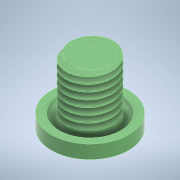
# Autodesk Inventor part: screw_oring
Saved by Autodesk Inventor 2022 (Build 260153000, 153)
## iProperties
Created: 2022-10-25
Part Number: screw_oring
Material: Ogólny
Document SubType Name: Modeling
Designer: kosak
Density: 1 g/cm^3
Appearance: Gładki — ciemna zieleń leśna
Author: kosak
Autodesk Inventor part; units mm, degrees
ref_plane "YZ Plane" through (0, 0, 0) normal (1, 0, 0) x (0, 1, 0)
ref_plane "XZ Plane" through (0, 0, 0) normal (0, 1, 0) x (-1, 0, 0)
ref_plane "XY Plane" through (0, 0, 0) normal (0, 0, 1) x (1, 0, 0)
sketch "Szkic1" plane through (0, 0, 0) normal (0, 1, 0) x (-1, 0, 0)
  circle A0 centre (0, 0) radius 11.5
  dimension "d0" = 23
  constraints: 1 centre point, 1 coincident
  measures "d0" diameter of A0
extrude "Wyciągnięcie proste1" add sketch "Szkic1" along normal blind 4
sketch "Szkic2" plane through (0, 4, 0) normal (0, 1, 0) x (1, 0, 0)
  circle A0 centre (0, 0) radius 6.85
  circle A1 centre (0, 0) radius 9.15
  dimension "d3" = 13.7
  dimension "d4" = 18.3
  constraints: 2 centre point, 2 coincident
  measures "d3" diameter of A0
  measures "d4" diameter of A1
extrude "Wyciągnięcie proste2" cut sketch "Szkic2" against normal blind 1.5
sketch "Szkic3" plane through (0, 4, 0) normal (0, 1, 0) x (1, 0, 0)
  circle A0 centre (0, 0) radius 7
  dimension "d8" = 14
  constraints: 1 centre point, 1 coincident
  measures "d8" diameter of A0
extrude "Wyciągnięcie proste3" add sketch "Szkic3" along normal blind 15
thread "Gwint1" size "M14x2" class "6g" standard "ANSI Metric M Profile" full length
full round fillet "Zaokrąglenie pełne3" first side at (9.1203, 3, 0.7363) centre faces at (8.2947, 2.5, 0.7299) second side at (6.8278, 3, 0.5512)
sketch "Szkic5" plane through (0, 19, 0) normal (1, 0, 0) x (0, 0, 1)
  line L0 (7, 0) -> (7, 15)
  line L1 (7, 15) -> (5.5171, 15)
  line L2 (5.5171, 15) -> (5.5171, 0)
  line L3 (5.5171, 0) -> (7, 0)
  line L4 (0, -6.4171) -> (0, 23.2362) projected
  constraints: 8 end point
revolve "Obrót1" cut sketch "Szkic5" angle 360 about axis through (0, 19, 0) along (0, -1, 0)
sketch "Szkic6" plane through (0, 19, 0) normal (1, 0, 0) x (0, 0, 1)
  line L0 (7, 0) -> (7, 15)
  line L1 (7, 15) -> (5.5171, 15)
  line L2 (5.5171, 15) -> (5.5171, 0)
  line L3 (5.5171, 0) -> (7, 0)
  line L4 (0, -6.4171) -> (0, 23.2362) projected
  constraints: 8 end point
revolve "Obrót2" add sketch "Szkic6" angle 360 about axis through (0, 19, 0) along (0, -1, 0) separate body
sketch "Szkic4" plane through (0, 19, 0) normal (-1, 0, 0) x (0, -1, 0)
  line L0 (-1.1668, -5.6184) -> (-1.0001, -5.6184) construction
  line L1 (0.1666, -6.899) -> (-0.0001, -7.2192) construction
  line L2 (-2.0001, -7.2192) -> (-2.1668, -6.899) construction
  line L3 (-0.8334, -5.6184) -> (-1.0001, -5.2982) construction
  line L4 (-1.0001, -5.2982) -> (-1.1668, -5.6184) construction
  line L5 (-2.0001, -7.2192) -> (-1.8334, -6.899) construction
  line L6 (-0.8334, -5.6184) -> (-0.1668, -6.899)
  line L7 (-2.1668, -6.899) -> (-1.8334, -6.899) construction
  arc A0 (-2.1668, -6.899) -> (-2.0001, -7.0002) centre (-2.0001, -6.8123) ccw construction
  line L8 (0.1666, -6.899) -> (-0.1668, -6.899) construction
  line L9 (-2.0001, -7.2192) -> (-2.0001, -6.899) construction
  line L10 (-0.0001, -7.2192) -> (-0.0001, -6.899) construction
  line L11 (-1.0001, -5.2982) -> (-1.0001, -5.5172) construction
  line L12 (-2.0001, -7.0002) -> (-0.0001, -7.0002)
  arc A1 (-2.0001, -7.0002) -> (-1.8334, -6.899) centre (-2.0001, -6.8123) ccw
  line L13 (-0.1668, -6.899) -> (-0.0001, -7.2192) construction
  line L14 (-1.8334, -6.899) -> (-1.1668, -5.6184)
  line L15 (-0.0001, -0.0002) -> (-0.0001, 0.0177)
  line L16 (-0.0001, 0.0177) -> (-0.0001, -0.0002)
  line L17 (-0.0001, -0.0002) -> (0.0334, -0.0002)
  arc A2 (-0.1668, -6.899) -> (-0.0001, -7.0002) centre (-0.0001, -6.8123) ccw
  arc A3 (-0.0001, -7.0002) -> (0.1666, -6.899) centre (-0.0001, -6.8123) ccw construction
  arc A4 (-1.0001, -5.5172) -> (-1.1668, -5.6184) centre (-1.0001, -5.7051) ccw
  arc A5 (-0.8334, -5.6184) -> (-1.0001, -5.5172) centre (-1.0001, -5.7051) ccw
  line L18 (-1.0001, -5.5172) -> (-1.0001, -5.6184) construction
  line L19 (-1.0001, -5.6184) -> (-0.8334, -5.6184) construction
  dimension "d13" = 55
  dimension "d14" = 0.3202
  dimension "d15" = 0.3202
  dimension "Szkic4_ThreadOffset" = 0
  dimension "Szkic4_MajorRadius" = 7
  dimension "d18" = 2
  dimension "Szkic4_MinorRadius" = 5.5171
  constraints: 40 end point, 12 point on circle, 10 parallel, 8 tangent, 6 centre point, 6 collinear, 2 midpoint, 2 point on line, 1 horizontal, 1 perpendicular, 3 other
  measures "d13" angle of L6 L14
  measures "d14" distance of L3.end L0.end
  measures "d15" distance of L1.end L10.end
  measures "Szkic4_ThreadOffset" distance between parallel lines of L15 L10
  measures "Szkic4_MajorRadius" distance from line of L12 L15.start
  measures "d18" distance from line of L1.end L9
  measures "Szkic4_MinorRadius" distance edge to line of A5 L17
coil "Zwój1" sketch "Szkic4" operation cut axis through (0, 19, 0) along (0, -1, 0) pitch 2.002 turns 9.490509 hand right bodies 2
equation "\"d13\" = d20"
equation "\"d14\" = 0.160083 * Szkic4_Pitch"
equation "\"d15\" = 0.160083 * Szkic4_Pitch"
equation "\"d18\" = Szkic4_Pitch"
equation "\"d20\" = 55deg"
equation "\"Szkic4_Pitch\" = 2"
